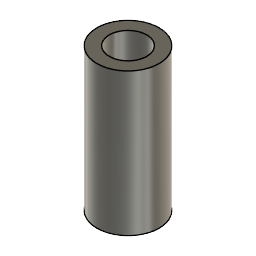
LegPivot (Autodesk Fusion 360 design; units mm, degrees)
part number: 2026-06-01-01-58-39-700
Autodesk Fusion 360 part; units mm, degrees
sketch "Sketch1" plane through (0, 0, 0) normal (0, 0, 1) x (1, 0, 0)
  circle A0 centre (0, 0) radius 5.2
  circle A1 centre (0, 0) radius 8.65
  dimension "d2" = 10.4
  dimension "d3" = 17.3
  constraint coincident A0.centre A1.centre
  measures "d2" diameter of A0
  measures "d3" diameter of A1
extrude "Extrude1" add sketch "Sketch1" along normal blind 39.7
equation "Tolerance = 0.1 mm"
equation "d2 = 10 mm + 4 * Tolerance"
equation "d3 = 17.5 mm - 2 * Tolerance"
